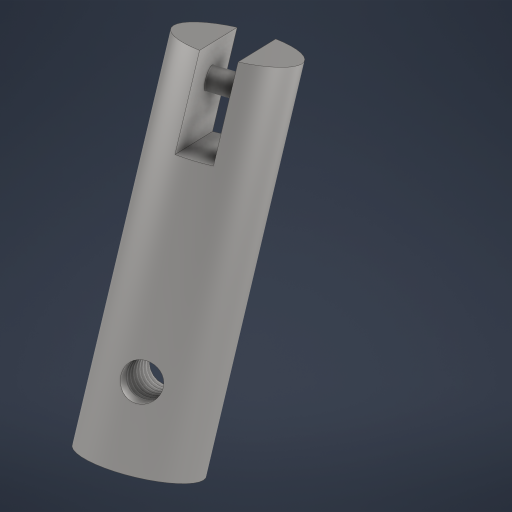
# Autodesk Inventor part: barrel_hinge-female
Saved by Autodesk Inventor 2023 (Build 270158000, 158)
## iProperties
Created: 2022-04-22
Part Number: barrel_hinge-female
Material: Stainless Steel
Document SubType Name: Sheet Metal
Designer: LigasN
Density: 8 g/cm^3
Sheet Metal Rule: Default
Appearance: Stainless - Brushed
Title: Stand construction
Subject: NormalMapScanner
Author: LigasN
Comments: https://github.com/LigasN/NormalMapScanner/discussions/14
Autodesk Inventor part; units mm, degrees
ref_plane "YZ Plane" through (0, 0, 0) normal (1, 0, 0) x (0, 1, 0)
ref_plane "XZ Plane" through (0, 0, 0) normal (0, 1, 0) x (-1, 0, 0)
sketch "Sketch1" plane through (0, 0, 0) normal (0, 1, 0) x (-1, 0, 0)
  circle A0 centre (0, 0) radius 5
  dimension "d0" = 10
  constraints: 1 centre point, 1 coincident
  measures "d0" diameter of A0
extrude "Extrusion1" add sketch "Sketch1" along normal blind 32
sketch "Sketch2" plane through (0, 32, 0) normal (0, 1, 0) x (1, 0, 0)
  line L0 (-1.5, 5) -> (1.5, 5)
  line L1 (1.5, 5) -> (1.5, -5)
  line L2 (1.5, -5) -> (-1.5, -5)
  line L3 (-1.5, -5) -> (-1.5, 5)
  point P0 (0, 0)
  point P1 (-1.5, 0)
  point P2 (0, 5)
  dimension "d3" = 3
  dimension "d4" = 10
  constraints: 8 end point, 2 midpoint, 1 horizontal alignment, 1 vertical alignment
  measures "d3" distance of L0.start L0.end
  measures "d4" distance of L2.end L0.start
extrude "Extrusion2" cut sketch "Sketch2" against normal blind 8
sketch "Sketch3" plane through (1.5, 32, -4.7697) normal (-1, 0, 0) x (0, 0, 1)
  circle A0 centre (4.7697, -3) radius 1
  line L0 (9.5394, 0) -> (0, 0) projected
  point P0 (4.7697, -32)
  point P1 (4.7697, 0)
  dimension "d7" = 2
  dimension "d8" = 3
  constraints: 1 centre point, 1 midpoint, 1 vertical alignment
  measures "d7" diameter of A0
  measures "d8" distance from line of L0 A0.centre
extrude "Extrusion3" add sketch "Sketch3" along normal blind 3
ref_plane "Work Plane1" through (0, 0, -5) normal (0, 0, 1) x (1, 0, 0)
sketch "Sketch5" plane through (0, 0, -5) normal (0, 0, 1) x (1, 0, 0)
  point P0 (0, 0)
  point P1 (0, 7)
  dimension "d14" = 7
  constraints: 1 vertical alignment
  measures "d14" distance of point (0, 0) point (0, 7)
hole "Hole1" at (0, 7, -5) direction (0, 0, 1) diameter 3.302 end through all countersink diameter 8 countersink angle 90 thread size "8-32 UNC" class "2B" standard "ANSI Unified Screw Threads"
equation "\"d20\" = Thickness"
equation "\"BendRadius\" = Thickness"
equation "\"BendReliefWidth\" = Thickness"
equation "\"BendReliefDepth\" = 0.5 * Thickness"
equation "\"CornerReliefSize\" = 4 * Thickness"
equation "\"MinimumRemnant\" = 2 * Thickness"
equation "\"TransitionRadius\" = BendRadius"
equation "\"JacobiRadiusSize\" = BendRadius"
equation "\"GapSize\" = Thickness"
equation "\"Thickness\" = 3.048"
